Autodesk Inventor part; units mm, degrees
(part 5 of 9)
sketch "Sketch34" plane through (0, 0, 0) normal (1, 0, 0) x (0, 0, -1)
  circle A0 centre (-11.1125, -19.2474) radius 2.2479 projected
  circle A1 centre (-11.1125, 19.2474) radius 2.2479 projected
  circle A2 centre (22.225, 0) radius 2.2479 projected
  circle A3 centre (11.1125, 19.2474) radius 2.2479 projected
  circle A4 centre (-22.225, 0) radius 2.2479 projected
  circle A5 centre (11.1125, -19.2474) radius 2.2479 projected
  circle A6 centre (-148.682, -242.899) radius 2.5527 projected
  circle A7 centre (-116.932, -39.699) radius 2.5527 projected
  circle A8 centre (-148.682, -39.699) radius 2.5527 projected
  circle A9 centre (-186.782, -179.399) radius 2.5527 projected
  circle A10 centre (143.418, 63.5) radius 2.5527 projected
  circle A11 centre (-8.982, 63.5) radius 2.5527 projected
  circle A12 centre (-59.782, 63.5) radius 2.5527 projected
  circle A13 centre (67.218, 63.5) radius 2.5527 projected
  circle A14 centre (-186.782, -242.899) radius 2.5527 projected
  circle A15 centre (-186.782, -39.699) radius 2.5527 projected
  circle A16 centre (-148.682, -179.399) radius 2.5527 projected
  circle A17 centre (-116.932, -179.399) radius 2.5527 projected
  circle A18 centre (-116.932, -242.899) radius 2.5527 projected
  circle A19 centre (145.0649, -242.899) radius 2.5527 projected
  circle A20 centre (97.9437, -242.899) radius 2.5527 projected
  circle A21 centre (70.3186, -242.899) radius 2.5527 projected
  circle A22 centre (122.2368, -242.899) radius 2.5527 projected
  circle A23 centre (145.0649, -113.4346) radius 2.5527 projected
  line L0 (-35.2916, -227.024) -> (-35.2916, -53.975) projected
  arc A24 (-32.1166, -50.8) -> (-35.2916, -53.975) centre (-32.1166, -53.975) ccw projected
  line L1 (-32.1166, -50.8) -> (42.0514, -50.8) projected
  arc A25 (74.705, -62.6849) -> (42.0514, -50.8) centre (42.0514, -101.6) ccw projected
  line L2 (74.705, -62.6849) -> (142.7266, -119.7618) projected
  line L3 (114.3, -156.3452) -> (114.3, -116.9566) projected
  arc A26 (113.8746, -157.9327) -> (114.3, -156.3452) centre (111.125, -156.3452) ccw projected
  line L4 (73.0682, -228.6115) -> (113.8746, -157.9327) projected
  arc A27 (70.3186, -230.199) -> (73.0682, -228.6115) centre (70.3186, -227.024) ccw projected
  line L5 (-32.1166, -230.199) -> (70.3186, -230.199) projected
  arc A28 (-35.2916, -227.024) -> (-32.1166, -230.199) centre (-32.1166, -227.024) ccw projected
  circle A29 centre (160.7915, -118.9794) radius 2.5527 projected
  circle A30 centre (-85.7798, -94.9817) radius 2.4892 projected
  circle A31 centre (-110.3931, -99.2933) radius 2.4892 projected
  circle A32 centre (-101.8395, -50.0579) radius 2.4892 projected
  circle A33 centre (-124.2369, -62.8574) radius 2.4892 projected
  circle A34 centre (-110.6604, -51.6228) radius 2.4892 projected
  circle A35 centre (-93.2858, -99.3592) radius 2.4892 projected
  circle A36 centre (-93.0185, -51.5569) radius 2.4892 projected
  circle A37 centre (-101.8395, -100.8579) radius 2.4892 projected
  circle A38 centre (-80.2428, -88.2574) radius 2.4892 projected
  circle A39 centre (239.2356, -31.496) radius 3.3782 projected
  circle A40 centre (223.7295, 90.3926) radius 3.3782 projected
  circle A41 centre (239.2356, 31.496) radius 3.3782 projected
  circle A42 centre (221.404, -95.9477) radius 3.3782 projected
  line L6 (149.831, -89.2272) -> (89.9434, -38.9755) projected
  arc A43 (88.9, -36.7379) -> (89.9434, -38.9755) centre (91.821, -36.7379) ccw projected
  line L7 (88.9, -36.7379) -> (88.9, -15.621) projected
  arc A44 (91.821, -12.7) -> (88.9, -15.621) centre (91.821, -15.621) ccw projected
  line L8 (91.821, -12.7) -> (174.1799, -12.7) projected
  arc A45 (177.0893, -15.8819) -> (174.1799, -12.7) centre (174.1799, -15.621) ccw projected
  arc A46 (154.2425, -88.4425) -> (177.0893, -15.8819) centre (0, 0) ccw projected
  arc A47 (149.831, -89.2272) -> (154.2425, -88.4425) centre (151.7086, -86.9895) ccw projected
  line L9 (88.9, -0.254) -> (88.9, 0.254) projected
  arc A48 (91.821, 3.175) -> (88.9, 0.254) centre (91.821, 0.254) ccw projected
  line L10 (91.821, 3.175) -> (174.4218, 3.175) projected
  arc A49 (177.3428, 0.254) -> (174.4218, 3.175) centre (174.4218, 0.254) ccw projected
  line L11 (177.3428, 0.254) -> (177.3428, -0.254) projected
  arc A50 (174.4218, -3.175) -> (177.3428, -0.254) centre (174.4218, -0.254) ccw projected
  line L12 (174.4218, -3.175) -> (91.821, -3.175) projected
  arc A51 (88.9, -0.254) -> (91.821, -3.175) centre (91.821, -0.254) ccw projected
  arc A52 (177.0893, 15.8819) -> (169.6939, 53.0738) centre (0, 0) ccw projected
  arc A53 (174.1799, 12.7) -> (177.0893, 15.8819) centre (174.1799, 15.621) ccw projected
  line L13 (174.1799, 12.7) -> (91.821, 12.7) projected
  arc A54 (88.9, 15.621) -> (91.821, 12.7) centre (91.821, 15.621) ccw projected
  line L14 (88.9, 15.621) -> (88.9, 17.1891) projected
  arc A55 (90.5865, 19.8364) -> (88.9, 17.1891) centre (91.821, 17.1891) ccw projected
  line L15 (90.5865, 19.8364) -> (165.6716, 54.8492) projected
  arc A56 (169.6939, 53.0738) -> (165.6716, 54.8492) centre (166.9061, 52.2019) ccw projected
  arc A57 (180.8991, -105.7674) -> (203.0448, 51.8076) centre (0, 0) ccw projected
  arc A58 (204.8485, 54.889) -> (203.0448, 51.8076) centre (205.5059, 52.4355) ccw projected
  line L16 (204.8485, 54.889) -> (206.0753, 55.2177) projected
  arc A59 (209.1938, 53.3924) -> (206.0753, 55.2177) centre (206.7327, 52.7643) ccw projected
  arc A60 (186.3731, -108.9857) -> (209.1938, 53.3924) centre (0, 0) ccw projected
  arc A61 (182.8723, -109.8807) -> (186.3731, -108.9857) centre (184.1805, -107.7035) ccw projected
  line L17 (182.8723, -109.8807) -> (181.7836, -109.2266) projected
  arc A62 (180.8991, -105.7674) -> (181.7836, -109.2266) centre (183.0918, -107.0494) ccw projected
  arc A63 (159.1231, -92.6879) -> (178.5072, 45.237) centre (0, 0) ccw projected
  arc A64 (180.312, 48.3145) -> (178.5072, 45.237) centre (180.9694, 45.861) ccw projected
  line L18 (180.312, 48.3145) -> (181.5388, 48.6432) projected
  arc A65 (184.6584, 46.8139) -> (181.5388, 48.6432) centre (182.1962, 46.1897) ccw projected
  arc A66 (164.6013, -95.8992) -> (184.6584, 46.8139) centre (0, 0) ccw projected
  arc A67 (161.0985, -96.7977) -> (164.6013, -95.8992) centre (162.4067, -94.6205) ccw projected
  line L19 (161.0985, -96.7977) -> (160.0098, -96.1436) projected
  arc A68 (159.1231, -92.6879) -> (160.0098, -96.1436) centre (161.3179, -93.9664) ccw projected
  line L20 (171.9854, -103.3393) -> (170.8967, -102.6851) projected
  arc A69 (170.0112, -99.2275) -> (170.8967, -102.6851) centre (172.2049, -100.5079) ccw projected
  arc A70 (170.0112, -99.2275) -> (190.7761, 48.5222) centre (0, 0) ccw projected
  arc A71 (192.5803, 51.6017) -> (190.7761, 48.5222) centre (193.2377, 49.1483) ccw projected
  line L21 (192.5803, 51.6017) -> (193.8071, 51.9305) projected
  arc A72 (196.9261, 50.1033) -> (193.8071, 51.9305) centre (194.4645, 49.477) ccw projected
  arc A73 (175.4872, -102.4426) -> (196.9261, 50.1033) centre (0, 0) ccw projected
  arc A74 (171.9854, -103.3393) -> (175.4872, -102.4426) centre (173.2936, -101.1621) ccw projected
  circle A75 centre (187.962, 68.4126) radius 2.5527 projected
  circle A76 centre (0, 0) radius 13.335 projected
  circle A77 centre (-193.0957, -164.2646) radius 2.4892 projected
  circle A78 centre (-180.6733, -167.7222) radius 2.4892 projected
  circle A79 centre (-168.1768, -164.3742) radius 2.4892 projected
  circle A80 centre (-173.4354, -117.9041) radius 2.4892 projected
  circle A81 centre (-186.8225, -117.6771) radius 2.4892 projected
  circle A82 centre (-193.0957, -120.1058) radius 2.4892 projected
  circle A83 centre (-180.1195, -116.9252) radius 2.4892 projected
  circle A84 centre (-167.2175, -120.5501) radius 2.4892 projected
  circle A85 centre (-174.2102, -166.8866) radius 2.4892 projected
  circle A86 centre (-187.1176, -166.8269) radius 2.4892 projected
  line L22 (-85.3603, 16.259) -> (-85.3603, 6.734) projected
  arc A87 (-90.1228, 1.9715) -> (-85.3603, 6.734) centre (-90.1228, 6.734) ccw projected
  line L23 (-90.1228, 1.9715) -> (-121.8728, 1.9715) projected
  arc A88 (-126.6353, 6.734) -> (-121.8728, 1.9715) centre (-121.8728, 6.734) ccw projected
  line L24 (-126.6353, 6.734) -> (-126.6353, 16.259) projected
  line L25 (-126.6353, 16.259) -> (-132.3503, 16.259) projected
  arc A89 (-132.3503, 22.609) -> (-132.3503, 16.259) centre (-132.3503, 19.434) ccw projected
  line L26 (-132.3503, 22.609) -> (-126.6353, 22.609) projected
  line L27 (-126.6353, 22.609) -> (-126.6353, 32.134) projected
  arc A90 (-121.8728, 36.8965) -> (-126.6353, 32.134) centre (-121.8728, 32.134) ccw projected
  line L28 (-121.8728, 36.8965) -> (-90.1228, 36.8965) projected
  arc A91 (-85.3603, 32.134) -> (-90.1228, 36.8965) centre (-90.1228, 32.134) ccw projected
  line L29 (-85.3603, 32.134) -> (-85.3603, 22.609) projected
  line L30 (-85.3603, 22.609) -> (-79.6453, 22.609) projected
  arc A92 (-79.6453, 16.259) -> (-79.6453, 22.609) centre (-79.6453, 19.434) ccw projected
  line L31 (-79.6453, 16.259) -> (-85.3603, 16.259) projected
  line L32 (-117.9165, 59.8835) -> (-80.5978, 59.8835) projected
  arc A93 (-80.5978, 54.7781) -> (-80.5978, 59.8835) centre (-80.5978, 57.3308) ccw projected
  line L33 (-80.5978, 54.7781) -> (-123.0219, 54.7781) projected
  line L34 (-112.3478, -13.7765) -> (-99.6478, -13.7765) projected
  arc A94 (-99.6478, -18.8819) -> (-99.6478, -13.7765) centre (-99.6478, -16.3292) ccw projected
  line L35 (-99.6478, -18.8819) -> (-112.3478, -18.8819) projected
  arc A95 (-112.3478, -13.7765) -> (-112.3478, -18.8819) centre (-112.3478, -16.3292) ccw projected
  line L36 (-199.482, -255.599) -> (149.8274, -255.599) projected
  line L37 (194.4526, -163.563) -> (149.8274, -255.599) projected
  arc A96 (194.8736, -162.9119) -> (194.4526, -163.563) centre (197.3095, -164.9483) ccw projected
  arc A97 (194.8736, -162.9119) -> (235.5329, 95.0804) centre (0, 0) ccw projected
  arc A98 (235.5329, 95.0804) -> (218.389, 101.8364) centre (223.7562, 90.3263) ccw projected
  line L38 (218.389, 101.8364) -> (173.6183, 80.9596) projected
  arc A99 (152.1493, 76.2) -> (173.6183, 80.9596) centre (152.1493, 127) ccw projected
  line L39 (152.1493, 76.2) -> (-101.6, 76.2) projected
  line L40 (-101.6, 76.2) -> (-117.9165, 59.8835) projected
  line L41 (-199.482, -21.682) -> (-199.482, -255.599) projected
  line L42 (-101.6, 76.2) -> (-199.482, 76.2)
  line L43 (-199.482, 76.2) -> (-199.482, -21.682)
  line L44 (-101.6, 76.2) -> (152.1493, 76.2) projected
  line L45 (-199.482, -21.682) -> (-101.6, 76.2)
  line L46 (114.3, -116.9566) -> (142.7266, -119.7618) projected
  arc A100 (-99.6119, -84.758) -> (-99.4903, -84.728) centre (-101.8395, -75.4579) ccw projected
  circle A101 centre (-118.4334, -56.0666) radius 2.4892 projected
  arc A102 (-99.4903, -84.728) -> (-104.0551, -66.155) centre (-101.7058, -75.4251) ccw projected
  arc A103 (-99.7334, -84.7881) -> (-99.6119, -84.758) centre (-101.9731, -75.491) ccw projected
  arc A104 (-99.8547, -84.8183) -> (-99.7334, -84.7881) centre (-102.1066, -75.5241) ccw projected
  arc A105 (-104.4917, -66.2632) -> (-99.8547, -84.8183) centre (-102.2399, -75.5574) ccw projected
  arc A106 (-104.3463, -66.227) -> (-104.4917, -66.2632) centre (-102.1066, -75.5241) ccw projected
  arc A107 (-104.2008, -66.1909) -> (-104.3463, -66.227) centre (-101.9731, -75.491) ccw projected
  arc A108 (-104.0551, -66.155) -> (-104.2008, -66.1909) centre (-101.8395, -75.4579) ccw projected
  line L47 (-123.0219, 54.7781) -> (-199.482, -21.682) projected
  constraints: 6 end point, 1 horizontal, 1 perpendicular
extrude "Extrusion19" add sketch "Sketch34" against normal up to surface (3.175 mm away) contours L45 L43 L42 L40
sketch "Sketch35" plane through (0, 0, 0) normal (1, 0, 0) x (0, 0, -1)
  line L0 (-169.4924, -15.1474) -> (-144.4783, -19.5581)
  line L1 (-144.4783, -19.5581) -> (-134.003, 39.8505)
  line L2 (-134.003, 39.8505) -> (-159.0171, 44.2611)
  line L3 (-159.0171, 44.2611) -> (-169.4924, -15.1474)
  circle A0 centre (-11.1125, -19.2474) radius 2.2479 projected
  circle A1 centre (-11.1125, 19.2474) radius 2.2479 projected
  circle A2 centre (22.225, 0) radius 2.2479 projected
  circle A3 centre (11.1125, 19.2474) radius 2.2479 projected
  circle A4 centre (-22.225, 0) radius 2.2479 projected
  circle A5 centre (11.1125, -19.2474) radius 2.2479 projected
  circle A6 centre (-148.682, -242.899) radius 2.5527 projected
  circle A7 centre (-116.932, -39.699) radius 2.5527 projected
  circle A8 centre (-148.682, -39.699) radius 2.5527 projected
  circle A9 centre (-186.782, -179.399) radius 2.5527 projected
  circle A10 centre (143.418, 63.5) radius 2.5527 projected
  circle A11 centre (-8.982, 63.5) radius 2.5527 projected
  circle A12 centre (-59.782, 63.5) radius 2.5527 projected
  circle A13 centre (67.218, 63.5) radius 2.5527 projected
  circle A14 centre (-186.782, -242.899) radius 2.5527 projected
  circle A15 centre (-186.782, -39.699) radius 2.5527 projected
  circle A16 centre (-148.682, -179.399) radius 2.5527 projected
  circle A17 centre (-116.932, -179.399) radius 2.5527 projected
  circle A18 centre (-116.932, -242.899) radius 2.5527 projected
  circle A19 centre (145.0649, -242.899) radius 2.5527 projected
  circle A20 centre (97.9437, -242.899) radius 2.5527 projected
  circle A21 centre (70.3186, -242.899) radius 2.5527 projected
  circle A22 centre (122.2368, -242.899) radius 2.5527 projected
  circle A23 centre (145.0649, -113.4346) radius 2.5527 projected
  line L4 (-35.2916, -227.024) -> (-35.2916, -53.975) projected
  arc A24 (-32.1166, -50.8) -> (-35.2916, -53.975) centre (-32.1166, -53.975) ccw projected
  line L5 (-32.1166, -50.8) -> (42.0514, -50.8) projected
  arc A25 (74.705, -62.6849) -> (42.0514, -50.8) centre (42.0514, -101.6) ccw projected
  line L6 (74.705, -62.6849) -> (142.7266, -119.7618) projected
  line L7 (114.3, -156.3452) -> (114.3, -116.9566) projected
  arc A26 (113.8746, -157.9327) -> (114.3, -156.3452) centre (111.125, -156.3452) ccw projected
  line L8 (73.0682, -228.6115) -> (113.8746, -157.9327) projected
  arc A27 (70.3186, -230.199) -> (73.0682, -228.6115) centre (70.3186, -227.024) ccw projected
  line L9 (-32.1166, -230.199) -> (70.3186, -230.199) projected
  arc A28 (-35.2916, -227.024) -> (-32.1166, -230.199) centre (-32.1166, -227.024) ccw projected
  circle A29 centre (160.7915, -118.9794) radius 2.5527 projected
  circle A30 centre (-85.7798, -94.9817) radius 2.4892 projected
  circle A31 centre (-110.3931, -99.2933) radius 2.4892 projected
  circle A32 centre (-101.8395, -50.0579) radius 2.4892 projected
  circle A33 centre (-124.2369, -62.8574) radius 2.4892 projected
  circle A34 centre (-110.6604, -51.6228) radius 2.4892 projected
  circle A35 centre (-93.2858, -99.3592) radius 2.4892 projected
  circle A36 centre (-93.0185, -51.5569) radius 2.4892 projected
  circle A37 centre (-101.8395, -100.8579) radius 2.4892 projected
  circle A38 centre (-80.2428, -88.2574) radius 2.4892 projected
  circle A39 centre (239.2356, -31.496) radius 3.3782 projected
  circle A40 centre (223.7295, 90.3926) radius 3.3782 projected
  circle A41 centre (239.2356, 31.496) radius 3.3782 projected
  circle A42 centre (221.404, -95.9477) radius 3.3782 projected
  line L10 (149.831, -89.2272) -> (89.9434, -38.9755) projected
  arc A43 (88.9, -36.7379) -> (89.9434, -38.9755) centre (91.821, -36.7379) ccw projected
  line L11 (88.9, -36.7379) -> (88.9, -15.621) projected
  arc A44 (91.821, -12.7) -> (88.9, -15.621) centre (91.821, -15.621) ccw projected
  line L12 (91.821, -12.7) -> (174.1799, -12.7) projected
  arc A45 (177.0893, -15.8819) -> (174.1799, -12.7) centre (174.1799, -15.621) ccw projected
  arc A46 (154.2425, -88.4425) -> (177.0893, -15.8819) centre (0, 0) ccw projected
  arc A47 (149.831, -89.2272) -> (154.2425, -88.4425) centre (151.7086, -86.9895) ccw projected
  line L13 (88.9, -0.254) -> (88.9, 0.254) projected
  arc A48 (91.821, 3.175) -> (88.9, 0.254) centre (91.821, 0.254) ccw projected
  line L14 (91.821, 3.175) -> (174.4218, 3.175) projected
  arc A49 (177.3428, 0.254) -> (174.4218, 3.175) centre (174.4218, 0.254) ccw projected
  line L15 (177.3428, 0.254) -> (177.3428, -0.254) projected
  arc A50 (174.4218, -3.175) -> (177.3428, -0.254) centre (174.4218, -0.254) ccw projected
  line L16 (174.4218, -3.175) -> (91.821, -3.175) projected
  arc A51 (88.9, -0.254) -> (91.821, -3.175) centre (91.821, -0.254) ccw projected
  arc A52 (177.0893, 15.8819) -> (169.6939, 53.0738) centre (0, 0) ccw projected
  arc A53 (174.1799, 12.7) -> (177.0893, 15.8819) centre (174.1799, 15.621) ccw projected
  line L17 (174.1799, 12.7) -> (91.821, 12.7) projected
  arc A54 (88.9, 15.621) -> (91.821, 12.7) centre (91.821, 15.621) ccw projected
  line L18 (88.9, 15.621) -> (88.9, 17.1891) projected
  arc A55 (90.5865, 19.8364) -> (88.9, 17.1891) centre (91.821, 17.1891) ccw projected
  line L19 (90.5865, 19.8364) -> (165.6716, 54.8492) projected
  arc A56 (169.6939, 53.0738) -> (165.6716, 54.8492) centre (166.9061, 52.2019) ccw projected
  arc A57 (180.8991, -105.7674) -> (203.0448, 51.8076) centre (0, 0) ccw projected
  arc A58 (204.8485, 54.889) -> (203.0448, 51.8076) centre (205.5059, 52.4355) ccw projected
  line L20 (204.8485, 54.889) -> (206.0753, 55.2177) projected
  arc A59 (209.1938, 53.3924) -> (206.0753, 55.2177) centre (206.7327, 52.7643) ccw projected
  arc A60 (186.3731, -108.9857) -> (209.1938, 53.3924) centre (0, 0) ccw projected
  arc A61 (182.8723, -109.8807) -> (186.3731, -108.9857) centre (184.1805, -107.7035) ccw projected
  line L21 (182.8723, -109.8807) -> (181.7836, -109.2266) projected
  arc A62 (180.8991, -105.7674) -> (181.7836, -109.2266) centre (183.0918, -107.0494) ccw projected
  arc A63 (159.1231, -92.6879) -> (178.5072, 45.237) centre (0, 0) ccw projected
  arc A64 (180.312, 48.3145) -> (178.5072, 45.237) centre (180.9694, 45.861) ccw projected
  line L22 (180.312, 48.3145) -> (181.5388, 48.6432) projected
  arc A65 (184.6584, 46.8139) -> (181.5388, 48.6432) centre (182.1962, 46.1897) ccw projected
  arc A66 (164.6013, -95.8992) -> (184.6584, 46.8139) centre (0, 0) ccw projected
  arc A67 (161.0985, -96.7977) -> (164.6013, -95.8992) centre (162.4067, -94.6205) ccw projected
  line L23 (161.0985, -96.7977) -> (160.0098, -96.1436) projected
  arc A68 (159.1231, -92.6879) -> (160.0098, -96.1436) centre (161.3179, -93.9664) ccw projected
  line L24 (171.9854, -103.3393) -> (170.8967, -102.6851) projected
  arc A69 (170.0112, -99.2275) -> (170.8967, -102.6851) centre (172.2049, -100.5079) ccw projected
  arc A70 (170.0112, -99.2275) -> (190.7761, 48.5222) centre (0, 0) ccw projected
  arc A71 (192.5803, 51.6017) -> (190.7761, 48.5222) centre (193.2377, 49.1483) ccw projected
  line L25 (192.5803, 51.6017) -> (193.8071, 51.9305) projected
  arc A72 (196.9261, 50.1033) -> (193.8071, 51.9305) centre (194.4645, 49.477) ccw projected
  arc A73 (175.4872, -102.4426) -> (196.9261, 50.1033) centre (0, 0) ccw projected
  arc A74 (171.9854, -103.3393) -> (175.4872, -102.4426) centre (173.2936, -101.1621) ccw projected
  circle A75 centre (187.962, 68.4126) radius 2.5527 projected
  circle A76 centre (0, 0) radius 13.335 projected
  circle A77 centre (-193.0957, -164.2646) radius 2.4892 projected
  circle A78 centre (-180.6733, -167.7222) radius 2.4892 projected
  circle A79 centre (-168.1768, -164.3742) radius 2.4892 projected
  circle A80 centre (-173.4354, -117.9041) radius 2.4892 projected
  circle A81 centre (-186.8225, -117.6771) radius 2.4892 projected
  circle A82 centre (-193.0957, -120.1058) radius 2.4892 projected
  circle A83 centre (-180.1195, -116.9252) radius 2.4892 projected
  circle A84 centre (-167.2175, -120.5501) radius 2.4892 projected
  circle A85 centre (-174.2102, -166.8866) radius 2.4892 projected
  circle A86 centre (-187.1176, -166.8269) radius 2.4892 projected
  line L26 (-85.3603, 16.259) -> (-85.3603, 6.734) projected
  arc A87 (-90.1228, 1.9715) -> (-85.3603, 6.734) centre (-90.1228, 6.734) ccw projected
  line L27 (-90.1228, 1.9715) -> (-121.8728, 1.9715) projected
  arc A88 (-126.6353, 6.734) -> (-121.8728, 1.9715) centre (-121.8728, 6.734) ccw projected
  line L28 (-126.6353, 6.734) -> (-126.6353, 16.259) projected
  line L29 (-126.6353, 16.259) -> (-132.3503, 16.259) projected
  arc A89 (-132.3503, 22.609) -> (-132.3503, 16.259) centre (-132.3503, 19.434) ccw projected
  line L30 (-132.3503, 22.609) -> (-126.6353, 22.609) projected
  line L31 (-126.6353, 22.609) -> (-126.6353, 32.134) projected
  arc A90 (-121.8728, 36.8965) -> (-126.6353, 32.134) centre (-121.8728, 32.134) ccw projected
  line L32 (-121.8728, 36.8965) -> (-90.1228, 36.8965) projected
  arc A91 (-85.3603, 32.134) -> (-90.1228, 36.8965) centre (-90.1228, 32.134) ccw projected
  line L33 (-85.3603, 32.134) -> (-85.3603, 22.609) projected
  line L34 (-85.3603, 22.609) -> (-79.6453, 22.609) projected
  arc A92 (-79.6453, 16.259) -> (-79.6453, 22.609) centre (-79.6453, 19.434) ccw projected
  line L35 (-79.6453, 16.259) -> (-85.3603, 16.259) projected
  line L36 (-117.9165, 59.8835) -> (-80.5978, 59.8835) projected
  arc A93 (-80.5978, 54.7781) -> (-80.5978, 59.8835) centre (-80.5978, 57.3308) ccw projected
  line L37 (-80.5978, 54.7781) -> (-123.0219, 54.7781) projected
  line L38 (-112.3478, -13.7765) -> (-99.6478, -13.7765) projected
  arc A94 (-99.6478, -18.8819) -> (-99.6478, -13.7765) centre (-99.6478, -16.3292) ccw projected
  line L39 (-99.6478, -18.8819) -> (-112.3478, -18.8819) projected
  arc A95 (-112.3478, -13.7765) -> (-112.3478, -18.8819) centre (-112.3478, -16.3292) ccw projected
  line L40 (-199.482, -255.599) -> (149.8274, -255.599) projected
  line L41 (194.4526, -163.563) -> (149.8274, -255.599) projected
  arc A96 (194.8736, -162.9119) -> (194.4526, -163.563) centre (197.3095, -164.9483) ccw projected
  arc A97 (194.8736, -162.9119) -> (235.5329, 95.0804) centre (0, 0) ccw projected
  arc A98 (235.5329, 95.0804) -> (218.389, 101.8364) centre (223.7562, 90.3263) ccw projected
  line L42 (218.389, 101.8364) -> (173.6183, 80.9596) projected
  arc A99 (152.1493, 76.2) -> (173.6183, 80.9596) centre (152.1493, 127) ccw projected
  line L43 (152.1493, 76.2) -> (-199.482, 76.2) projected
  line L44 (-199.482, 76.2) -> (-199.482, -255.599) projected
  line L45 (-199.482, 76.2) -> (-199.482, -255.599) projected
  line L46 (-135.6494, -24.3388) -> (-123.52, 44.45)
  line L47 (114.3, -116.9566) -> (142.7266, -119.7618) projected
  arc A100 (-99.6119, -84.758) -> (-99.4903, -84.728) centre (-101.8395, -75.4579) ccw projected
  circle A101 centre (-118.4334, -56.0666) radius 2.4892 projected
  arc A102 (-99.4903, -84.728) -> (-104.0551, -66.155) centre (-101.7058, -75.4251) ccw projected
  arc A103 (-99.7334, -84.7881) -> (-99.6119, -84.758) centre (-101.9731, -75.491) ccw projected
  arc A104 (-99.8547, -84.8183) -> (-99.7334, -84.7881) centre (-102.1066, -75.5241) ccw projected
  arc A105 (-104.4917, -66.2632) -> (-99.8547, -84.8183) centre (-102.2399, -75.5574) ccw projected
  arc A106 (-104.3463, -66.227) -> (-104.4917, -66.2632) centre (-102.1066, -75.5241) ccw projected
  arc A107 (-104.2008, -66.1909) -> (-104.3463, -66.227) centre (-101.9731, -75.491) ccw projected
  arc A108 (-104.0551, -66.155) -> (-104.2008, -66.1909) centre (-101.8395, -75.4579) ccw projected
  line L48 (-123.0219, 54.7781) -> (-117.9165, 59.8835) projected
  dimension "d558" = 25.4
  dimension "d559" = 60.325
  dimension "d561" = 3.175
  dimension "d562" = 69.85
  dimension "d563" = 9.525
  dimension "d564" = 15.3602
  dimension "d574" = 31.75
  dimension "d575" = 75.962
  dimension "d576" = 10
  constraints: 10 end point, 3 parallel, 1 perpendicular, 1 other
  measures "d558" distance of L0.start L0.end
  measures "d559" distance of L2.end L0.start
  measures "d561" distance from line of L46.start L0
  measures "d562" distance of L46.end L46.start
  measures "d563" distance from line of L1 L46.start
  measures "d564" vertical distance of A8.centre L46.start
  measures "d574" distance from line of L43 L46.end
  measures "d575" distance from line of L44 L46.end
  measures "d576" angle of L44 L3
hole "Limelight Hole" at (0, 44.45, 123.52) direction (-1, 0, 0) diameter 4.9784 end through all clearance for "Flat Head Machine Screw (82)" size "#10" standard "Ansi Unified Screw Threads"
sketch "Sketch36" plane through (0, 0, 0) normal (1, 0, 0) x (0, 0, -1)
  circle A0 centre (-123.52, 44.45) radius 2.4892 projected
  circle A1 centre (-11.1125, -19.2474) radius 2.2479 projected
  circle A2 centre (-11.1125, 19.2474) radius 2.2479 projected
  circle A3 centre (22.225, 0) radius 2.2479 projected
  circle A4 centre (11.1125, 19.2474) radius 2.2479 projected
  circle A5 centre (-22.225, 0) radius 2.2479 projected
  circle A6 centre (11.1125, -19.2474) radius 2.2479 projected
  circle A7 centre (-148.682, -242.899) radius 2.5527 projected
  circle A8 centre (-116.932, -39.699) radius 2.5527 projected
  circle A9 centre (-148.682, -39.699) radius 2.5527 projected
  circle A10 centre (-186.782, -179.399) radius 2.5527 projected
  circle A11 centre (143.418, 63.5) radius 2.5527 projected
  circle A12 centre (-8.982, 63.5) radius 2.5527 projected
  circle A13 centre (-59.782, 63.5) radius 2.5527 projected
  circle A14 centre (67.218, 63.5) radius 2.5527 projected
  circle A15 centre (-186.782, -242.899) radius 2.5527 projected
  circle A16 centre (-186.782, -39.699) radius 2.5527 projected
  circle A17 centre (-148.682, -179.399) radius 2.5527 projected
  circle A18 centre (-116.932, -179.399) radius 2.5527 projected
  circle A19 centre (-116.932, -242.899) radius 2.5527 projected
  circle A20 centre (145.0649, -242.899) radius 2.5527 projected
  circle A21 centre (97.9437, -242.899) radius 2.5527 projected
  circle A22 centre (70.3186, -242.899) radius 2.5527 projected
  circle A23 centre (122.2368, -242.899) radius 2.5527 projected
  circle A24 centre (145.0649, -113.4346) radius 2.5527 projected
  line L0 (-35.2916, -227.024) -> (-35.2916, -53.975) projected
  arc A25 (-32.1166, -50.8) -> (-35.2916, -53.975) centre (-32.1166, -53.975) ccw projected
  line L1 (-32.1166, -50.8) -> (42.0514, -50.8) projected
  arc A26 (74.705, -62.6849) -> (42.0514, -50.8) centre (42.0514, -101.6) ccw projected
  line L2 (74.705, -62.6849) -> (142.7266, -119.7618) projected
  line L3 (114.3, -156.3452) -> (114.3, -116.9566) projected
  arc A27 (113.8746, -157.9327) -> (114.3, -156.3452) centre (111.125, -156.3452) ccw projected
  line L4 (73.0682, -228.6115) -> (113.8746, -157.9327) projected
  arc A28 (70.3186, -230.199) -> (73.0682, -228.6115) centre (70.3186, -227.024) ccw projected
  line L5 (-32.1166, -230.199) -> (70.3186, -230.199) projected
  arc A29 (-35.2916, -227.024) -> (-32.1166, -230.199) centre (-32.1166, -227.024) ccw projected
  circle A30 centre (160.7915, -118.9794) radius 2.5527 projected
  circle A31 centre (-85.7798, -94.9817) radius 2.4892 projected
  circle A32 centre (-110.3931, -99.2933) radius 2.4892 projected
  circle A33 centre (-101.8395, -50.0579) radius 2.4892 projected
  circle A34 centre (-124.2369, -62.8574) radius 2.4892 projected
  circle A35 centre (-110.6604, -51.6228) radius 2.4892 projected
  circle A36 centre (-93.2858, -99.3592) radius 2.4892 projected
  circle A37 centre (-93.0185, -51.5569) radius 2.4892 projected
  circle A38 centre (-101.8395, -100.8579) radius 2.4892 projected
  circle A39 centre (-80.2428, -88.2574) radius 2.4892 projected
  circle A40 centre (239.2356, -31.496) radius 3.3782 projected
  circle A41 centre (223.7295, 90.3926) radius 3.3782 projected
  circle A42 centre (239.2356, 31.496) radius 3.3782 projected
  circle A43 centre (221.404, -95.9477) radius 3.3782 projected
  line L6 (149.831, -89.2272) -> (89.9434, -38.9755) projected
  arc A44 (88.9, -36.7379) -> (89.9434, -38.9755) centre (91.821, -36.7379) ccw projected
  line L7 (88.9, -36.7379) -> (88.9, -15.621) projected
  arc A45 (91.821, -12.7) -> (88.9, -15.621) centre (91.821, -15.621) ccw projected
  line L8 (91.821, -12.7) -> (174.1799, -12.7) projected
  arc A46 (177.0893, -15.8819) -> (174.1799, -12.7) centre (174.1799, -15.621) ccw projected
  arc A47 (154.2425, -88.4425) -> (177.0893, -15.8819) centre (0, 0) ccw projected
  arc A48 (149.831, -89.2272) -> (154.2425, -88.4425) centre (151.7086, -86.9895) ccw projected
  line L9 (88.9, -0.254) -> (88.9, 0.254) projected
  arc A49 (91.821, 3.175) -> (88.9, 0.254) centre (91.821, 0.254) ccw projected
  line L10 (91.821, 3.175) -> (174.4218, 3.175) projected
  arc A50 (177.3428, 0.254) -> (174.4218, 3.175) centre (174.4218, 0.254) ccw projected
  line L11 (177.3428, 0.254) -> (177.3428, -0.254) projected
  arc A51 (174.4218, -3.175) -> (177.3428, -0.254) centre (174.4218, -0.254) ccw projected
  line L12 (174.4218, -3.175) -> (91.821, -3.175) projected
  arc A52 (88.9, -0.254) -> (91.821, -3.175) centre (91.821, -0.254) ccw projected
  arc A53 (177.0893, 15.8819) -> (169.6939, 53.0738) centre (0, 0) ccw projected
  arc A54 (174.1799, 12.7) -> (177.0893, 15.8819) centre (174.1799, 15.621) ccw projected
  line L13 (174.1799, 12.7) -> (91.821, 12.7) projected
  arc A55 (88.9, 15.621) -> (91.821, 12.7) centre (91.821, 15.621) ccw projected
  line L14 (88.9, 15.621) -> (88.9, 17.1891) projected
  arc A56 (90.5865, 19.8364) -> (88.9, 17.1891) centre (91.821, 17.1891) ccw projected
  line L15 (90.5865, 19.8364) -> (165.6716, 54.8492) projected
  arc A57 (169.6939, 53.0738) -> (165.6716, 54.8492) centre (166.9061, 52.2019) ccw projected
  arc A58 (180.8991, -105.7674) -> (203.0448, 51.8076) centre (0, 0) ccw projected
  arc A59 (204.8485, 54.889) -> (203.0448, 51.8076) centre (205.5059, 52.4355) ccw projected
  line L16 (204.8485, 54.889) -> (206.0753, 55.2177) projected
  arc A60 (209.1938, 53.3924) -> (206.0753, 55.2177) centre (206.7327, 52.7643) ccw projected
  arc A61 (186.3731, -108.9857) -> (209.1938, 53.3924) centre (0, 0) ccw projected
  arc A62 (182.8723, -109.8807) -> (186.3731, -108.9857) centre (184.1805, -107.7035) ccw projected
  line L17 (182.8723, -109.8807) -> (181.7836, -109.2266) projected
  arc A63 (180.8991, -105.7674) -> (181.7836, -109.2266) centre (183.0918, -107.0494) ccw projected
  arc A64 (159.1231, -92.6879) -> (178.5072, 45.237) centre (0, 0) ccw projected
  arc A65 (180.312, 48.3145) -> (178.5072, 45.237) centre (180.9694, 45.861) ccw projected
  line L18 (180.312, 48.3145) -> (181.5388, 48.6432) projected
  arc A66 (184.6584, 46.8139) -> (181.5388, 48.6432) centre (182.1962, 46.1897) ccw projected
  arc A67 (164.6013, -95.8992) -> (184.6584, 46.8139) centre (0, 0) ccw projected
  arc A68 (161.0985, -96.7977) -> (164.6013, -95.8992) centre (162.4067, -94.6205) ccw projected
  line L19 (161.0985, -96.7977) -> (160.0098, -96.1436) projected
  arc A69 (159.1231, -92.6879) -> (160.0098, -96.1436) centre (161.3179, -93.9664) ccw projected
  line L20 (171.9854, -103.3393) -> (170.8967, -102.6851) projected
  arc A70 (170.0112, -99.2275) -> (170.8967, -102.6851) centre (172.2049, -100.5079) ccw projected
  arc A71 (170.0112, -99.2275) -> (190.7761, 48.5222) centre (0, 0) ccw projected
  arc A72 (192.5803, 51.6017) -> (190.7761, 48.5222) centre (193.2377, 49.1483) ccw projected
  line L21 (192.5803, 51.6017) -> (193.8071, 51.9305) projected
  arc A73 (196.9261, 50.1033) -> (193.8071, 51.9305) centre (194.4645, 49.477) ccw projected
  arc A74 (175.4872, -102.4426) -> (196.9261, 50.1033) centre (0, 0) ccw projected
  arc A75 (171.9854, -103.3393) -> (175.4872, -102.4426) centre (173.2936, -101.1621) ccw projected
  circle A76 centre (187.962, 68.4126) radius 2.5527 projected
  circle A77 centre (0, 0) radius 13.335 projected
  circle A78 centre (-193.0957, -164.2646) radius 2.4892 projected
  circle A79 centre (-180.6733, -167.7222) radius 2.4892 projected
  circle A80 centre (-168.1768, -164.3742) radius 2.4892 projected
  circle A81 centre (-173.4354, -117.9041) radius 2.4892 projected
  circle A82 centre (-186.8225, -117.6771) radius 2.4892 projected
  circle A83 centre (-193.0957, -120.1058) radius 2.4892 projected
  circle A84 centre (-180.1195, -116.9252) radius 2.4892 projected
  circle A85 centre (-167.2175, -120.5501) radius 2.4892 projected
  circle A86 centre (-174.2102, -166.8866) radius 2.4892 projected
  circle A87 centre (-187.1176, -166.8269) radius 2.4892 projected
  line L22 (-85.3603, 16.259) -> (-85.3603, 6.734) projected
  arc A88 (-90.1228, 1.9715) -> (-85.3603, 6.734) centre (-90.1228, 6.734) ccw projected
  line L23 (-90.1228, 1.9715) -> (-121.8728, 1.9715) projected
  arc A89 (-126.6353, 6.734) -> (-121.8728, 1.9715) centre (-121.8728, 6.734) ccw projected
  line L24 (-126.6353, 6.734) -> (-126.6353, 16.259) projected
  line L25 (-126.6353, 16.259) -> (-132.3503, 16.259) projected
  arc A90 (-132.3503, 22.609) -> (-132.3503, 16.259) centre (-132.3503, 19.434) ccw projected
  line L26 (-132.3503, 22.609) -> (-126.6353, 22.609) projected
  line L27 (-126.6353, 22.609) -> (-126.6353, 32.134) projected
  arc A91 (-121.8728, 36.8965) -> (-126.6353, 32.134) centre (-121.8728, 32.134) ccw projected
  line L28 (-121.8728, 36.8965) -> (-90.1228, 36.8965) projected
  arc A92 (-85.3603, 32.134) -> (-90.1228, 36.8965) centre (-90.1228, 32.134) ccw projected
  line L29 (-85.3603, 32.134) -> (-85.3603, 22.609) projected
  line L30 (-85.3603, 22.609) -> (-79.6453, 22.609) projected
  arc A93 (-79.6453, 16.259) -> (-79.6453, 22.609) centre (-79.6453, 19.434) ccw projected
  line L31 (-79.6453, 16.259) -> (-85.3603, 16.259) projected
  line L32 (-117.9165, 59.8835) -> (-80.5978, 59.8835) projected
  arc A94 (-80.5978, 54.7781) -> (-80.5978, 59.8835) centre (-80.5978, 57.3308) ccw projected
  line L33 (-80.5978, 54.7781) -> (-123.0219, 54.7781) projected
  line L34 (-112.3478, -13.7765) -> (-99.6478, -13.7765) projected
  arc A95 (-99.6478, -18.8819) -> (-99.6478, -13.7765) centre (-99.6478, -16.3292) ccw projected
  line L35 (-99.6478, -18.8819) -> (-112.3478, -18.8819) projected
  arc A96 (-112.3478, -13.7765) -> (-112.3478, -18.8819) centre (-112.3478, -16.3292) ccw projected
  line L36 (-199.482, -255.599) -> (149.8274, -255.599) projected
  line L37 (194.4526, -163.563) -> (149.8274, -255.599) projected
  arc A97 (194.8736, -162.9119) -> (194.4526, -163.563) centre (197.3095, -164.9483) ccw projected
  arc A98 (194.8736, -162.9119) -> (235.5329, 95.0804) centre (0, 0) ccw projected
  arc A99 (235.5329, 95.0804) -> (218.389, 101.8364) centre (223.7562, 90.3263) ccw projected
  line L38 (218.389, 101.8364) -> (173.6183, 80.9596) projected
  arc A100 (152.1493, 76.2) -> (173.6183, 80.9596) centre (152.1493, 127) ccw projected
  line L39 (152.1493, 76.2) -> (-199.482, 76.2) projected
  line L40 (-199.482, 76.2) -> (-199.482, -255.599) projected
  arc A101 (-133.1907, -24.7273) -> (-170.2968, -7.4245) centre (-123.52, 44.45) ccw
  line L41 (-123.52, 44.45) -> (-135.2171, -21.8874)
  line L42 (-123.52, 44.45) -> (-166.8187, -7.1514)
  arc A102 (-166.8187, -7.1514) -> (-170.0188, -10.965) centre (-168.4187, -9.0582) ccw
  arc A103 (-136.0816, -26.7902) -> (-135.2171, -21.8874) centre (-135.6494, -24.3388) ccw
  arc A104 (-166.8187, -7.1514) -> (-135.2171, -21.8874) centre (-123.52, 44.45) ccw
  arc A105 (-170.0188, -10.965) -> (-136.0816, -26.7902) centre (-123.52, 44.45) ccw
  line L43 (114.3, -116.9566) -> (142.7266, -119.7618) projected
  arc A106 (-99.6119, -84.758) -> (-99.4903, -84.728) centre (-101.8395, -75.4579) ccw projected
  circle A107 centre (-118.4334, -56.0666) radius 2.4892 projected
  arc A108 (-99.4903, -84.728) -> (-104.0551, -66.155) centre (-101.7058, -75.4251) ccw projected
  arc A109 (-99.7334, -84.7881) -> (-99.6119, -84.758) centre (-101.9731, -75.491) ccw projected
  arc A110 (-99.8547, -84.8183) -> (-99.7334, -84.7881) centre (-102.1066, -75.5241) ccw projected
  arc A111 (-104.4917, -66.2632) -> (-99.8547, -84.8183) centre (-102.2399, -75.5574) ccw projected
  arc A112 (-104.3463, -66.227) -> (-104.4917, -66.2632) centre (-102.1066, -75.5241) ccw projected
  arc A113 (-104.2008, -66.1909) -> (-104.3463, -66.227) centre (-101.9731, -75.491) ccw projected
  arc A114 (-104.0551, -66.155) -> (-104.2008, -66.1909) centre (-101.8395, -75.4579) ccw projected
  line L44 (-123.0219, 54.7781) -> (-117.9165, 59.8835) projected
  dimension "d584" = 139.7
  dimension "d585" = 10
  dimension "d586" = 40
  dimension "d587" = 4.9784
  constraints: 14 point on circle, 5 centre point, 4 end point, 2 concentric, 2 tangent, 1 coincident, 1 equal radius
  measures "d584" diameter of A101
  measures "d585" angle of L40 L41
  measures "d586" angle of L40 L42
  measures "d587" diameter of A102
extrude "Limelight Slot" cut sketch "Sketch36" against normal through all contours A104 A103 A105 A102
fillet "Fillet10" radius 3.175 7 edges at (-1.5875, 22.609, 126.6353) (-1.5875, 16.259, 126.6353) (-1.5875, 22.609, 85.3603) (-1.5875, 16.259, 85.3603) (-1.5875, -255.599, -149.8274) (-1.5875, -255.599, 199.482) (-1.5875, 76.2, 199.482)
sketch "Sketch37" plane through (0, 0, 0) normal (1, 0, 0) x (0, 0, -1)
  arc A0 (-196.307, 76.2) -> (-199.482, 73.025) centre (-196.307, 73.025) ccw projected
  line L0 (-199.482, 73.025) -> (-199.482, -252.424) projected
  arc A1 (-199.482, -252.424) -> (-196.307, -255.599) centre (-196.307, -252.424) ccw projected
  line L1 (-196.307, -255.599) -> (147.8383, -255.599) projected
  arc A2 (147.8383, -255.599) -> (150.6952, -253.8092) centre (147.8383, -252.424) ccw projected
  line L2 (194.4526, -163.563) -> (150.6952, -253.8092) projected
  arc A3 (194.8736, -162.9119) -> (194.4526, -163.563) centre (197.3095, -164.9483) ccw projected
  arc A4 (194.8736, -162.9119) -> (235.5329, 95.0804) centre (0, 0) ccw projected
  arc A5 (235.5329, 95.0804) -> (218.389, 101.8364) centre (223.7562, 90.3263) ccw projected
  line L3 (218.389, 101.8364) -> (173.6183, 80.9596) projected
  arc A6 (152.1493, 76.2) -> (173.6183, 80.9596) centre (152.1493, 127) ccw projected
  line L4 (152.1493, 76.2) -> (-196.307, 76.2) projected
  arc A7 (-166.8187, -7.1514) -> (-170.0188, -10.965) centre (-168.4187, -9.0582) ccw projected
  arc A8 (-166.8187, -7.1514) -> (-135.2171, -21.8874) centre (-123.52, 44.45) ccw projected
  arc A9 (-136.0816, -26.7902) -> (-135.2171, -21.8874) centre (-135.6494, -24.3388) ccw projected
  arc A10 (-170.0188, -10.965) -> (-136.0816, -26.7902) centre (-123.52, 44.45) ccw projected
  circle A11 centre (-123.52, 44.45) radius 2.4892 projected
  circle A12 centre (-11.1125, -19.2474) radius 2.2479 projected
  circle A13 centre (-11.1125, 19.2474) radius 2.2479 projected
  circle A14 centre (22.225, 0) radius 2.2479 projected
  circle A15 centre (11.1125, 19.2474) radius 2.2479 projected
  circle A16 centre (-22.225, 0) radius 2.2479 projected
  circle A17 centre (11.1125, -19.2474) radius 2.2479 projected
  circle A18 centre (-148.682, -242.899) radius 2.5527 projected
  circle A19 centre (-116.932, -39.699) radius 2.5527 projected
  circle A20 centre (-148.682, -39.699) radius 2.5527 projected
  circle A21 centre (-186.782, -179.399) radius 2.5527 projected
  circle A22 centre (143.418, 63.5) radius 2.5527 projected
  circle A23 centre (-8.982, 63.5) radius 2.5527 projected
  circle A24 centre (-59.782, 63.5) radius 2.5527 projected
  circle A25 centre (67.218, 63.5) radius 2.5527 projected
  circle A26 centre (-186.782, -242.899) radius 2.5527 projected
  circle A27 centre (-186.782, -39.699) radius 2.5527 projected
  circle A28 centre (-148.682, -179.399) radius 2.5527 projected
  circle A29 centre (-116.932, -179.399) radius 2.5527 projected
  circle A30 centre (-116.932, -242.899) radius 2.5527 projected
  circle A31 centre (145.0649, -242.899) radius 2.5527 projected
  circle A32 centre (97.9437, -242.899) radius 2.5527 projected
  circle A33 centre (70.3186, -242.899) radius 2.5527 projected
  circle A34 centre (122.2368, -242.899) radius 2.5527 projected
  circle A35 centre (145.0649, -113.4346) radius 2.5527 projected
  line L5 (-35.2916, -227.024) -> (-35.2916, -53.975) projected
  arc A36 (-32.1166, -50.8) -> (-35.2916, -53.975) centre (-32.1166, -53.975) ccw projected
  line L6 (-32.1166, -50.8) -> (42.0514, -50.8) projected
  arc A37 (74.705, -62.6849) -> (42.0514, -50.8) centre (42.0514, -101.6) ccw projected
  line L7 (74.705, -62.6849) -> (142.7266, -119.7618) projected
  line L8 (114.3, -156.3452) -> (114.3, -116.9566) projected
  arc A38 (113.8746, -157.9327) -> (114.3, -156.3452) centre (111.125, -156.3452) ccw projected
  line L9 (73.0682, -228.6115) -> (113.8746, -157.9327) projected
  arc A39 (70.3186, -230.199) -> (73.0682, -228.6115) centre (70.3186, -227.024) ccw projected
  line L10 (-32.1166, -230.199) -> (70.3186, -230.199) projected
  arc A40 (-35.2916, -227.024) -> (-32.1166, -230.199) centre (-32.1166, -227.024) ccw projected
  circle A41 centre (160.7915, -118.9794) radius 2.5527 projected
  circle A42 centre (-85.7798, -94.9817) radius 2.4892 projected
  circle A43 centre (-110.3931, -99.2933) radius 2.4892 projected
  circle A44 centre (-101.8395, -50.0579) radius 2.4892 projected
  circle A45 centre (-124.2369, -62.8574) radius 2.4892 projected
  circle A46 centre (-110.6604, -51.6228) radius 2.4892 projected
  circle A47 centre (-93.2858, -99.3592) radius 2.4892 projected
  circle A48 centre (-93.0185, -51.5569) radius 2.4892 projected
  circle A49 centre (-101.8395, -100.8579) radius 2.4892 projected
  circle A50 centre (-80.2428, -88.2574) radius 2.4892 projected
  circle A51 centre (239.2356, -31.496) radius 3.3782 projected
  circle A52 centre (223.7295, 90.3926) radius 3.3782 projected
  circle A53 centre (239.2356, 31.496) radius 3.3782 projected
  circle A54 centre (221.404, -95.9477) radius 3.3782 projected
  line L11 (149.831, -89.2272) -> (89.9434, -38.9755) projected
  arc A55 (88.9, -36.7379) -> (89.9434, -38.9755) centre (91.821, -36.7379) ccw projected
  line L12 (88.9, -36.7379) -> (88.9, -15.621) projected
  arc A56 (91.821, -12.7) -> (88.9, -15.621) centre (91.821, -15.621) ccw projected
  line L13 (91.821, -12.7) -> (174.1799, -12.7) projected
  arc A57 (177.0893, -15.8819) -> (174.1799, -12.7) centre (174.1799, -15.621) ccw projected
  arc A58 (154.2425, -88.4425) -> (177.0893, -15.8819) centre (0, 0) ccw projected
  arc A59 (149.831, -89.2272) -> (154.2425, -88.4425) centre (151.7086, -86.9895) ccw projected
  line L14 (88.9, -0.254) -> (88.9, 0.254) projected
  arc A60 (91.821, 3.175) -> (88.9, 0.254) centre (91.821, 0.254) ccw projected
  line L15 (91.821, 3.175) -> (174.4218, 3.175) projected
  arc A61 (177.3428, 0.254) -> (174.4218, 3.175) centre (174.4218, 0.254) ccw projected
  line L16 (177.3428, 0.254) -> (177.3428, -0.254) projected
  arc A62 (174.4218, -3.175) -> (177.3428, -0.254) centre (174.4218, -0.254) ccw projected
  line L17 (174.4218, -3.175) -> (91.821, -3.175) projected
  arc A63 (88.9, -0.254) -> (91.821, -3.175) centre (91.821, -0.254) ccw projected
  arc A64 (177.0893, 15.8819) -> (169.6939, 53.0738) centre (0, 0) ccw projected
  arc A65 (174.1799, 12.7) -> (177.0893, 15.8819) centre (174.1799, 15.621) ccw projected
  line L18 (174.1799, 12.7) -> (91.821, 12.7) projected
  arc A66 (88.9, 15.621) -> (91.821, 12.7) centre (91.821, 15.621) ccw projected
  line L19 (88.9, 15.621) -> (88.9, 17.1891) projected
  arc A67 (90.5865, 19.8364) -> (88.9, 17.1891) centre (91.821, 17.1891) ccw projected
  line L20 (90.5865, 19.8364) -> (165.6716, 54.8492) projected
  arc A68 (169.6939, 53.0738) -> (165.6716, 54.8492) centre (166.9061, 52.2019) ccw projected
  arc A69 (180.8991, -105.7674) -> (203.0448, 51.8076) centre (0, 0) ccw projected
  arc A70 (204.8485, 54.889) -> (203.0448, 51.8076) centre (205.5059, 52.4355) ccw projected
  line L21 (204.8485, 54.889) -> (206.0753, 55.2177) projected
  arc A71 (209.1938, 53.3924) -> (206.0753, 55.2177) centre (206.7327, 52.7643) ccw projected
  arc A72 (186.3731, -108.9857) -> (209.1938, 53.3924) centre (0, 0) ccw projected
  arc A73 (182.8723, -109.8807) -> (186.3731, -108.9857) centre (184.1805, -107.7035) ccw projected
  line L22 (182.8723, -109.8807) -> (181.7836, -109.2266) projected
  arc A74 (180.8991, -105.7674) -> (181.7836, -109.2266) centre (183.0918, -107.0494) ccw projected
  arc A75 (159.1231, -92.6879) -> (178.5072, 45.237) centre (0, 0) ccw projected
  arc A76 (180.312, 48.3145) -> (178.5072, 45.237) centre (180.9694, 45.861) ccw projected
  line L23 (180.312, 48.3145) -> (181.5388, 48.6432) projected
  arc A77 (184.6584, 46.8139) -> (181.5388, 48.6432) centre (182.1962, 46.1897) ccw projected
  arc A78 (164.6013, -95.8992) -> (184.6584, 46.8139) centre (0, 0) ccw projected
  arc A79 (161.0985, -96.7977) -> (164.6013, -95.8992) centre (162.4067, -94.6205) ccw projected
  line L24 (161.0985, -96.7977) -> (160.0098, -96.1436) projected
  arc A80 (159.1231, -92.6879) -> (160.0098, -96.1436) centre (161.3179, -93.9664) ccw projected
  line L25 (171.9854, -103.3393) -> (170.8967, -102.6851) projected
  arc A81 (170.0112, -99.2275) -> (170.8967, -102.6851) centre (172.2049, -100.5079) ccw projected
  arc A82 (170.0112, -99.2275) -> (190.7761, 48.5222) centre (0, 0) ccw projected
  arc A83 (192.5803, 51.6017) -> (190.7761, 48.5222) centre (193.2377, 49.1483) ccw projected
  line L26 (192.5803, 51.6017) -> (193.8071, 51.9305) projected
  arc A84 (196.9261, 50.1033) -> (193.8071, 51.9305) centre (194.4645, 49.477) ccw projected
  arc A85 (175.4872, -102.4426) -> (196.9261, 50.1033) centre (0, 0) ccw projected
  arc A86 (171.9854, -103.3393) -> (175.4872, -102.4426) centre (173.2936, -101.1621) ccw projected
  circle A87 centre (187.962, 68.4126) radius 2.5527 projected
  circle A88 centre (0, 0) radius 13.335 projected
  circle A89 centre (-193.0957, -164.2646) radius 2.4892 projected
  circle A90 centre (-180.6733, -167.7222) radius 2.4892 projected
  circle A91 centre (-168.1768, -164.3742) radius 2.4892 projected
  circle A92 centre (-173.4354, -117.9041) radius 2.4892 projected
  circle A93 centre (-186.8225, -117.6771) radius 2.4892 projected
  circle A94 centre (-193.0957, -120.1058) radius 2.4892 projected
  circle A95 centre (-180.1195, -116.9252) radius 2.4892 projected
  circle A96 centre (-167.2175, -120.5501) radius 2.4892 projected
  circle A97 centre (-174.2102, -166.8866) radius 2.4892 projected
  circle A98 centre (-187.1176, -166.8269) radius 2.4892 projected
  arc A99 (-82.1853, 16.259) -> (-85.3603, 13.084) centre (-82.1853, 13.084) ccw projected
  line L27 (-85.3603, 13.084) -> (-85.3603, 6.734) projected
  arc A100 (-90.1228, 1.9715) -> (-85.3603, 6.734) centre (-90.1228, 6.734) ccw projected
  line L28 (-90.1228, 1.9715) -> (-121.8728, 1.9715) projected
  arc A101 (-126.6353, 6.734) -> (-121.8728, 1.9715) centre (-121.8728, 6.734) ccw projected
  line L29 (-126.6353, 6.734) -> (-126.6353, 13.084) projected
  arc A102 (-126.6353, 13.084) -> (-129.8103, 16.259) centre (-129.8103, 13.084) ccw projected
  line L30 (-129.8103, 16.259) -> (-132.3503, 16.259) projected
  arc A103 (-132.3503, 22.609) -> (-132.3503, 16.259) centre (-132.3503, 19.434) ccw projected
  line L31 (-132.3503, 22.609) -> (-129.8103, 22.609) projected
  arc A104 (-129.8103, 22.609) -> (-126.6353, 25.784) centre (-129.8103, 25.784) ccw projected
  line L32 (-126.6353, 25.784) -> (-126.6353, 32.134) projected
  arc A105 (-121.8728, 36.8965) -> (-126.6353, 32.134) centre (-121.8728, 32.134) ccw projected
  line L33 (-121.8728, 36.8965) -> (-90.1228, 36.8965) projected
  arc A106 (-85.3603, 32.134) -> (-90.1228, 36.8965) centre (-90.1228, 32.134) ccw projected
  line L34 (-85.3603, 32.134) -> (-85.3603, 25.784) projected
  arc A107 (-85.3603, 25.784) -> (-82.1853, 22.609) centre (-82.1853, 25.784) ccw projected
  line L35 (-82.1853, 22.609) -> (-79.6453, 22.609) projected
  arc A108 (-79.6453, 16.259) -> (-79.6453, 22.609) centre (-79.6453, 19.434) ccw projected
  line L36 (-79.6453, 16.259) -> (-82.1853, 16.259) projected
  line L37 (-117.9165, 59.8835) -> (-80.5978, 59.8835) projected
  arc A109 (-80.5978, 54.7781) -> (-80.5978, 59.8835) centre (-80.5978, 57.3308) ccw projected
  line L38 (-80.5978, 54.7781) -> (-123.0219, 54.7781) projected
  line L39 (-112.3478, -13.7765) -> (-99.6478, -13.7765) projected
  arc A110 (-99.6478, -18.8819) -> (-99.6478, -13.7765) centre (-99.6478, -16.3292) ccw projected
  line L40 (-99.6478, -18.8819) -> (-112.3478, -18.8819) projected
  arc A111 (-112.3478, -13.7765) -> (-112.3478, -18.8819) centre (-112.3478, -16.3292) ccw projected
  line L41 (114.3, -116.9566) -> (142.7266, -119.7618) projected
  arc A112 (-99.6119, -84.758) -> (-99.4903, -84.728) centre (-101.8395, -75.4579) ccw projected
  circle A113 centre (-118.4334, -56.0666) radius 2.4892 projected
  arc A114 (-99.4903, -84.728) -> (-104.0551, -66.155) centre (-101.7058, -75.4251) ccw projected
  arc A115 (-99.7334, -84.7881) -> (-99.6119, -84.758) centre (-101.9731, -75.491) ccw projected
  arc A116 (-99.8547, -84.8183) -> (-99.7334, -84.7881) centre (-102.1066, -75.5241) ccw projected
  arc A117 (-104.4917, -66.2632) -> (-99.8547, -84.8183) centre (-102.2399, -75.5574) ccw projected
  arc A118 (-104.3463, -66.227) -> (-104.4917, -66.2632) centre (-102.1066, -75.5241) ccw projected
  arc A119 (-104.2008, -66.1909) -> (-104.3463, -66.227) centre (-101.9731, -75.491) ccw projected
  arc A120 (-104.0551, -66.155) -> (-104.2008, -66.1909) centre (-101.8395, -75.4579) ccw projected
  line L42 (-123.0219, 54.7781) -> (-117.9165, 59.8835) projected
extrude "Extrusion21" add sketch "Sketch37" against normal up to surface (3.175 mm away) contours L5 A36 L6 A37 L7 L41 L8 A38 L9 A39 L10 A40